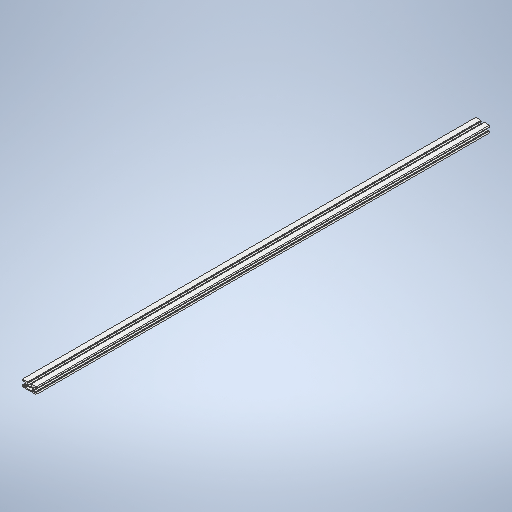
# Autodesk Inventor part: 15×30 3 slots profile_AST01503003
Saved by Autodesk Inventor 2025.2 (Build 292293000, 293)
## iProperties
Created: 2025-03-25
Part Number: 15×30 3 slots profile_AST01503003
Material: ABS plástico
Document SubType Name: Modeling
Designer: lucas
Density: 1.06 g/cm^3
Appearance: Suave - Branco
Author: lucas
Autodesk Inventor part; units mm, degrees
ref_plane "YZ Plane" through (0, 0, 0) normal (1, 0, 0) x (0, 1, 0)
ref_plane "XZ Plane" through (0, 0, 0) normal (0, 1, 0) x (-1, 0, 0)
ref_plane "XY Plane" through (0, 0, 0) normal (0, 0, 1) x (1, 0, 0)
sketch "Esboço3" plane through (0, 0, 0) normal (0, 0, 1) x (1, 0, 0)
  line L0 (-15, 15) -> (15, 15) construction
  line L1 (-3.1, 9) -> (3.1, 9) construction
  line L2 (-4.1, 7) -> (4.1, 7) construction
  line L3 (-3.1, 15) -> (3.1, 15) construction
  line L4 (-3.1, 9) -> (0, 9) construction
  line L5 (-3.1, 15) -> (-15, 15) construction
  line L6 (-3.1, 15) -> (-3.1, 13) construction
  line L7 (-3.1, 13) -> (-6.1, 13) construction
  line L8 (-6.1, 13) -> (-3.1, 9) construction
  line L9 (-15, 10.6) -> (-15, 4.4) construction
  line L10 (-15, 15) -> (-15, 10.6) construction
  line L11 (-15, 10.6) -> (-13, 10.6) construction
  line L12 (-13, 13.6) -> (-13, 10.6) construction
  line L13 (-8.8, 10.6) -> (-8.8, 4.4) construction
  line L14 (-13, 13.6) -> (-8.8, 10.6) construction
  line L15 (-15, 0) -> (0, 0)
  line L16 (-15, 0) -> (-15, 4.4) construction
  line L17 (-15, 4.4) -> (-13, 4.4) construction
  line L18 (-13, 4.4) -> (-13, 1.4) construction
  line L19 (-13, 1.4) -> (-8.8, 4.4) construction
  line L20 (-6.8, 10.6) -> (-4.1, 7) construction
  line L21 (-6.8, 10.6) -> (-6.8, 4.4) construction
  line L22 (-10.16, 2) -> (10.16, 2) construction
  line L23 (-10.16, 2) -> (-6.8, 4.4) construction
  line L24 (-10.16, 2) -> (0, 2) construction
  line L25 (-4.1, 7) -> (0, 7) construction
  line L26 (-3.1, 15) -> (-3.6, 15) construction
  line L27 (-3.6, 15) -> (-3.6, 14.5)
  line L28 (-3.6, 14.5) -> (-3.1, 14.5)
  line L29 (-3.1, 14.5) -> (-3.1, 15) construction
  line L30 (-3.1, 14.5) -> (-3.1, 13)
  line L31 (-3.6, 15) -> (-15, 15)
  line L32 (-15, 10.6) -> (-14.5, 10.6) construction
  line L33 (-14.5, 10.6) -> (-14.5, 11.1)
  line L34 (-14.5, 11.1) -> (-15, 11.1)
  line L35 (-15, 11.1) -> (-15, 10.6) construction
  line L36 (-15, 15) -> (-15, 11.1)
  line L37 (-14.5, 10.6) -> (-13, 10.6)
  line L38 (-15, 4.4) -> (-14.5, 4.4) construction
  line L39 (-14.5, 4.4) -> (-14.5, 3.9)
  line L40 (-14.5, 3.9) -> (-15, 3.9)
  line L41 (-15, 3.9) -> (-15, 4.4) construction
  line L42 (-15, 3.9) -> (-15, 0)
  line L43 (-14.5, 4.4) -> (-13, 4.4)
  arc A0 (-5.1, 13) -> (-5.5, 12.2) centre (-5.1, 12.5) ccw
  line L44 (-3.1, 13) -> (-5.1, 13)
  arc A1 (-3.25, 9.2) -> (-2.85, 9) centre (-2.85, 9.5) ccw
  line L45 (-3.25, 9.2) -> (-5.5, 12.2)
  line L46 (-2.85, 9) -> (0, 9)
  line L47 (-13, 12.628405) -> (-13, 10.6)
  line L48 (-13, 2.371595) -> (-13, 4.4)
  arc A2 (-12.209381, 13.035272) -> (-13, 12.628405) centre (-12.5, 12.628405) ccw
  arc A3 (-8.8, 10.6) -> (-8.8, 10.6) centre (-8.8, 10.6) ccw
  arc A4 (-9.009381, 4.250442) -> (-8.8, 4.657309) centre (-9.3, 4.657309) ccw
  arc A5 (-13, 2.371595) -> (-12.209381, 1.964728) centre (-12.5, 2.371595) ccw
  line L49 (-12.209381, 1.964728) -> (-9.009381, 4.250442)
  arc A6 (-8.8, 10.342691) -> (-9.009381, 10.749558) centre (-9.3, 10.342691) ccw
  line L50 (-12.209381, 13.035272) -> (-9.009381, 10.749558)
  line L51 (-8.8, 10.342691) -> (-8.8, 4.657309)
  arc A7 (-4.25, 7.2) -> (-3.85, 7) centre (-3.85, 7.5) ccw
  arc A8 (-5.9, 9.4) -> (-6.8, 9.1) centre (-6.3, 9.1) ccw
  arc A9 (-7.009381, 4.250442) -> (-6.8, 4.657309) centre (-7.3, 4.657309) ccw
  arc A10 (-8.890387, 2.906867) -> (-8.599767, 2) centre (-8.599767, 2.5) ccw
  line L52 (-4.25, 7.2) -> (-5.9, 9.4)
  line L53 (-6.8, 9.1) -> (-6.8, 4.657309)
  line L54 (-7.009381, 4.250442) -> (-8.890387, 2.906867)
  line L55 (-8.599767, 2) -> (0, 2)
  line L56 (-3.6, 15) -> (0, 15)
  line L57 (0, 15) -> (0, 9)
  line L58 (0, 9) -> (0, 7)
  line L59 (-3.85, 7) -> (0, 7)
  line L60 (0, 7) -> (0, 2)
  line L61 (0, 2) -> (0, 0)
  point P0 (-15, 7.5)
  point P1 (-8.8, 10.6)
  point P2 (-8.8, 7.5)
  point P3 (-6.8, 7.5)
  dimension "d33" = 15
  dimension "d34" = 6
  dimension "d35" = 30
  dimension "d36" = 2
  dimension "d37" = 6.2
  dimension "d38" = 2
  dimension "d39" = 3
  dimension "d40" = 6.2
  dimension "d41" = 2
  dimension "d43" = 3
  dimension "d44" = 2
  dimension "d45" = 2
  dimension "d46" = 2
  dimension "d47" = 0.5
  dimension "d52" = 0.5
  constraints: 124 end point, 26 tangent, 22 point on line, 20 point on circle, 16 collinear, 15 horizontal, 11 centre point, 10 vertical, 9 equal length, 9 equal radius, 9 vertical alignment, 8 midpoint, 8 parallel, 4 horizontal alignment, 4 perpendicular, 3 coincident, 3 coincident with centre
  measures "d33" distance from line of point (0, 0) L0
  measures "d34" distance between parallel lines of L0 L1
  measures "d35" distance of L0.start L0.end
  measures "d36" distance between parallel lines of L2 L1
  measures "d37" distance of L3.start L3.end
  measures "d38" distance of L3.start L6.end
  measures "d39" distance of L6.end L7.end
  measures "d40" distance of L9.start L9.end
  measures "d41" distance of L9.start L11.end
  measures "d43" distance of L12.start L11.end
  measures "d44" distance between parallel lines of L8 L20
  measures "d45" distance between parallel lines of L21 L13
  measures "d46" distance between parallel lines of L15 L22
  measures "d47" distance of L27.end L28.end
  measures "d52" radius of A0
sketch "Esboço3 outline for Extrusão1" plane through (0, 0, 0) normal (0, 0, 1) x (1, 0, 0)
  arc A0 (-4.25, 7.2) -> (-3.85, 7) centre (-3.85, 7.5) ccw
  line L0 (-5.9, 9.4) -> (-4.25, 7.2)
  arc A1 (-6.8, 9.1) -> (-5.9, 9.4) centre (-6.3, 9.1) cw
  line L1 (-6.8, 4.657309) -> (-6.8, 9.1)
  arc A2 (-7.009381, 4.250442) -> (-6.8, 4.657309) centre (-7.3, 4.657309) ccw
  line L2 (-8.890387, 2.906867) -> (-7.009381, 4.250442)
  arc A3 (-8.599767, 2) -> (-8.890387, 2.906867) centre (-8.599767, 2.5) cw
  line L3 (0, 2) -> (-8.599767, 2)
  line L4 (0, 0) -> (0, 2)
  line L5 (-15, 0) -> (0, 0)
  line L6 (-15, 3.9) -> (-15, 0)
  line L7 (-14.5, 3.9) -> (-15, 3.9)
  line L8 (-14.5, 4.4) -> (-14.5, 3.9)
  line L9 (-13, 4.4) -> (-14.5, 4.4)
  line L10 (-13, 2.371595) -> (-13, 4.4)
  arc A4 (-12.209381, 1.964728) -> (-13, 2.371595) centre (-12.5, 2.371595) cw
  line L11 (-9.009381, 4.250442) -> (-12.209381, 1.964728)
  arc A5 (-8.8, 4.657309) -> (-9.009381, 4.250442) centre (-9.3, 4.657309) cw
  line L12 (-8.8, 10.342691) -> (-8.8, 4.657309)
  arc A6 (-9.009381, 10.749558) -> (-8.8, 10.342691) centre (-9.3, 10.342691) cw
  line L13 (-12.209381, 13.035272) -> (-9.009381, 10.749558)
  arc A7 (-13, 12.628405) -> (-12.209381, 13.035272) centre (-12.5, 12.628405) cw
  line L14 (-13, 10.6) -> (-13, 12.628405)
  line L15 (-14.5, 10.6) -> (-13, 10.6)
  line L16 (-14.5, 11.1) -> (-14.5, 10.6)
  line L17 (-15, 11.1) -> (-14.5, 11.1)
  line L18 (-15, 15) -> (-15, 11.1)
  line L19 (-3.6, 15) -> (-15, 15)
  line L20 (-3.6, 14.5) -> (-3.6, 15)
  line L21 (-3.1, 14.5) -> (-3.6, 14.5)
  line L22 (-3.1, 13) -> (-3.1, 14.5)
  line L23 (-5.1, 13) -> (-3.1, 13)
  arc A8 (-5.5, 12.2) -> (-5.1, 13) centre (-5.1, 12.5) cw
  line L24 (-3.25, 9.2) -> (-5.5, 12.2)
  arc A9 (-2.85, 9) -> (-3.25, 9.2) centre (-2.85, 9.5) cw
  line L25 (0, 9) -> (-2.85, 9)
  line L26 (0, 7) -> (0, 9)
  line L27 (-3.85, 7) -> (0, 7)
extrude "Extrusão1" add sketch "Esboço3 outline for Extrusão1" along normal mid plane 1000
mirror "Espelhar1" about plane through (0, 0, 0) normal (1, 0, 0) of "Extrusão1"
